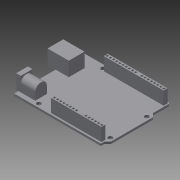
# Autodesk Inventor part: Arduino Uno
Saved by Autodesk Inventor 2015 (Build 190159000, 159)
## iProperties
Created: 2018-12-22
Part Number: Arduino Uno
Material: Типовые
Document SubType Name: Modeling
Designer: kostya
Density: 1 g/cm^3
Appearance: По умолчанию
Author: kostya
Autodesk Inventor part; units mm, degrees
ref_plane "YZ Plane" through (0, 0, 0) normal (1, 0, 0) x (0, 1, 0)
ref_plane "XZ Plane" through (0, 0, 0) normal (0, 1, 0) x (-1, 0, 0)
ref_plane "XY Plane" through (0, 0, 0) normal (0, 0, 1) x (1, 0, 0)
sketch "Эскиз1" plane through (0, 0, 0) normal (0, 0, 1) x (1, 0, 0)
  line L0 (-34.3, -26.6349) -> (31.8, -26.6349)
  line L1 (34.3, -21.3849) -> (34.3, 10.6851)
  line L2 (30.55, 26.6065) -> (-34.3, 26.6065)
  line L3 (-34.3, 26.6065) -> (-34.3, -26.6349)
  line L4 (-34.3, 26.6065) -> (-20.3, 26.6065) construction
  line L5 (-34.3, 26.6065) -> (16.5, 26.6065) construction
  line L6 (-34.3, 26.6065) -> (30.5, 26.6065) construction
  line L7 (34.3, 26.6065) -> (31.8, 26.6065) construction
  line L8 (-34.3, 26.6065) -> (-17, 26.6065) construction
  line L9 (-34.3, -26.6349) -> (-18.3, -26.6349) construction
  line L10 (-18.3, -26.6349) -> (-18.3, -25.4849) construction
  line L11 (-18.3, -25.4849) -> (-18.3, -22.2849) construction
  circle A0 centre (-18.3, -23.8849) radius 1.6
  line L12 (-17, 26.6065) -> (-17, 25.4565) construction
  line L13 (-17, 25.4565) -> (-17, 22.2565) construction
  circle A1 centre (-17, 23.8565) radius 1.6
  line L14 (34.3, -21.3849) -> (34.3, -19.1849) construction
  line L15 (34.3, -19.1849) -> (33.15, -19.1849) construction
  line L16 (33.15, -19.1849) -> (29.95, -19.1849) construction
  circle A2 centre (31.55, -19.1849) radius 1.6
  line L17 (31.55, -19.1849) -> (31.55, 8.7151) construction
  line L18 (31.55, 8.7151) -> (31.55, 10.3151) construction
  circle A3 centre (31.55, 8.7151) radius 1.6
  line L19 (-18.3, -23.8849) -> (34.3, -23.8849) construction
  line L20 (31.8, -23.8849) -> (34.3, -21.3849)
  line L21 (31.8, -23.8849) -> (34.3, -23.8849) construction
  line L22 (31.55, 10.3151) -> (31.55, 13.4351) construction
  line L23 (31.55, 13.4351) -> (34.3, 10.6851)
  line L24 (31.55, 13.4351) -> (35.4391, 13.4351) construction
  line L25 (31.55, 13.4351) -> (31.55, 25.6065)
  line L26 (31.8, -23.8849) -> (31.8, -26.6349)
  line L27 (31.55, 25.6065) -> (30.55, 26.6065)
  point P0 (0, 0)
  dimension "d0" = 68.6
  dimension "d7" = 17.3
  dimension "d8" = 16
  dimension "d9" = 1.15
  dimension "d10" = 3.2
  dimension "d11" = 1.15
  dimension "d12" = 3.2
  dimension "d13" = 4.7
  dimension "d14" = 1.15
  dimension "d15" = 3.2
  dimension "d18" = 27.9
  dimension "d19" = 1.6
  dimension "d20" = 45
  dimension "d21" = 3.12
  dimension "d22" = 45
  dimension "d25" = 53.2413
  constraints: 56 end point, 9 point on line, 6 horizontal, 4 vertical, 3 midpoint, 3 perpendicular, 3 vertical alignment, 2 parallel, 1 coincident, 1 equal length, 1 horizontal alignment, 8 other
  measures "d0" distance of L2.end L7.start
  measures "d7" distance of L2.end L8.end
  measures "d8" distance of L0.start L9.end
  measures "d9" distance of L9.end L10.end
  measures "d10" distance of L10.end L11.end
  measures "d11" distance of L8.end L12.end
  measures "d12" distance of L12.end L13.end
  measures "d13" distance of L19.end L14.end
  measures "d14" distance of L14.end L15.end
  measures "d15" distance of L15.end L16.end
  measures "d18" distance of L17.start L17.end
  measures "d19" distance of L17.end L18.end
  measures "d20" angle of L21 L20
  measures "d21" distance of L18.end L22.end
  measures "d22" angle of L23 L24
  measures "d25" distance of L7.end L0.end
extrude "Выдавливание1" add sketch "Эскиз1" along normal blind 1.6
sketch "Эскиз2" plane through (0, 0, 1.6) normal (0, 0, 1) x (1, 0, 0)
  circle A0 centre (31.55, 8.7151) radius 1.6 projected
  circle A1 centre (31.55, -19.1849) radius 1.6 projected
  circle A2 centre (-17, 23.8565) radius 1.6 projected
  circle A3 centre (-18.3, -23.8849) radius 1.6 projected
  line L0 (-34.3, -26.6349) -> (31.8, -26.6349) projected
  line L1 (31.8, -26.6349) -> (31.8, -23.8849) projected
  line L2 (31.8, -23.8849) -> (34.3, -21.3849) projected
  line L3 (34.3, -21.3849) -> (34.3, 10.6851) projected
  line L4 (34.3, 10.6851) -> (31.55, 13.4351) projected
  line L5 (31.55, 13.4351) -> (31.55, 25.6065) projected
  line L6 (31.55, 25.6065) -> (30.55, 26.6065) projected
  line L7 (30.55, 26.6065) -> (-34.3, 26.6065) projected
  line L8 (-34.3, 26.6065) -> (-34.3, -26.6349) projected
  line L9 (-34.3, 26.6065) -> (-34.3, 17.0065) construction
  line L10 (-34.3, 17.0065) -> (-40.5, 17.0065) construction
  line L11 (-40.5, 17.0065) -> (-40.5, 5.0065) construction
  line L12 (-40.5, 17.0065) -> (-24.3, 17.0065)
  line L13 (-24.3, 17.0065) -> (-24.3, 5.0065)
  line L14 (-24.3, 5.0065) -> (-40.5, 5.0065)
  line L15 (-40.5, 5.0065) -> (-40.5, 17.0065)
  line L16 (-34.3, -26.6349) -> (-34.3, -23.3349) construction
  line L17 (-34.3, 26.6065) -> (-34.3, -26.6349) construction
  line L18 (-34.3, -23.3349) -> (-36.1, -23.3349) construction
  line L19 (-36.1, -23.3349) -> (-36.1, -14.4349) construction
  line L20 (-36.1, -23.3349) -> (-21.6, -23.3349)
  line L21 (-21.6, -23.3349) -> (-21.6, -14.4349)
  line L22 (-21.6, -14.4349) -> (-36.1, -14.4349)
  line L23 (-36.1, -14.4349) -> (-36.1, -23.3349)
  point P0 (0, 0)
  dimension "d29" = 9.6
  dimension "d30" = 6.2
  dimension "d31" = 12
  dimension "d32" = 16.2
  dimension "d33" = 3.3
  dimension "d34" = 1.8
  dimension "d35" = 8.9
  dimension "d36" = 14.5
  constraints: 28 end point, 4 parallel, 4 perpendicular, 3 horizontal, 2 point on line, 1 vertical
  measures "d29" distance of L7.end L9.end
  measures "d30" distance of L9.end L10.end
  measures "d31" distance of L10.end L11.end
  measures "d32" distance of L13.end L14.end
  measures "d33" distance of L0.start L16.end
  measures "d34" distance of L16.end L18.end
  measures "d35" distance of L18.end L19.end
  measures "d36" distance of L22.end L21.end
extrude "Выдавливание2" add sketch "Эскиз2" along normal blind 10.9 contours L20 L23 L22 L8 | L8 L22 L21 L20 | L14 L15 L12 L8 | L8 L12 L13 L14
sketch "Эскиз3" plane through (-36.1, -23.3349, 1.6) normal (-1, 0, 0) x (0, 0, 1)
  line L0 (0, 8.9) -> (0, 0) projected
  line L1 (0, 0) -> (10.9, 0) projected
  line L2 (10.9, 8.9) -> (10.9, 0) projected
  line L3 (0, 8.9) -> (10.9, 8.9) projected
  line L4 (0, 8.9) -> (0, 0) projected
  line L5 (0, 4.45) -> (3.5, 4.45) construction
  line L6 (3.5, 4.45) -> (9.5, 4.45) construction
  circle A0 centre (6.5, 4.45) radius 3
  point P0 (-1.6, 23.3349)
  dimension "d39" = 3.5
  dimension "d40" = 6
  constraints: 4 end point, 2 horizontal, 2 midpoint, 1 horizontal alignment, 2 other
  measures "d39" distance of L5.start L5.end
  measures "d40" distance of L5.end L6.end
extrude "Выдавливание3" cut sketch "Эскиз3" against normal blind 9 contours A0
sketch "Эскиз4" plane through (-27.1, -18.8849, 8.1) normal (-1, 0, 0) x (0, 0, 1)
  circle A0 centre (0, 0) radius 0.5
  point P0 (-8.1, 18.8849)
  dimension "d43" = 1
  constraints: 1 centre point
  measures "d43" diameter of A0
extrude "Выдавливание4" add sketch "Эскиз4" along normal blind 9
fillet "Сопряжение1" radius 0.5 1 edges at (-36.1, -18.8849, 7.6)
sketch "Эскиз5" plane through (0, 0, 12.5) normal (0, 0, 1) x (1, 0, 0)
  line L0 (-36.1, -23.3349) -> (-21.6, -23.3349) projected
  line L1 (-21.6, -23.3349) -> (-21.6, -14.4349) projected
  line L2 (-21.6, -14.4349) -> (-36.1, -14.4349) projected
  line L3 (-36.1, -14.4349) -> (-36.1, -23.3349) projected
  line L4 (-36.1, -14.4349) -> (-32.6, -14.4349) construction
  line L5 (-21.6, -14.4349) -> (-36.1, -14.4349) construction
  line L6 (-32.6, -14.4349) -> (-32.6, -23.3349)
  line L7 (-36.1, -23.3349) -> (-21.6, -23.3349) projected
  line L8 (-36.1, -23.3349) -> (-32.6, -23.3349)
  line L9 (-36.1, -14.4349) -> (-36.1, -23.3349)
  line L10 (-36.1, -14.4349) -> (-32.6, -14.4349)
  point P0 (0, 0)
  dimension "d47" = 3.5
  constraints: 10 end point, 3 collinear, 2 point on line, 1 vertical
  measures "d47" distance of L2.end L4.end
extrude "Выдавливание5" cut sketch "Эскиз5" against normal blind 1 contours L6 L2 L1 L0
fillet "Сопряжение2" radius 4.25 2 edges at (-27.1, -23.3349, 11.5) (-27.1, -14.4349, 11.5)
sketch "Эскиз6" plane through (-40.5, 5.0065, 1.6) normal (-1, 0, 0) x (0, 0, 1)
  line L0 (0, 0) -> (0, 12) projected
  line L1 (0, 0) -> (10.9, 0) projected
  line L2 (10.9, 12) -> (10.9, 0) projected
  line L3 (0, 12) -> (10.9, 12) projected
  line L4 (10.9, 12) -> (10.9, 0) construction
  line L5 (10.9, 6) -> (0, 6) construction
  line L6 (0, 12) -> (0, 0) construction
  line L7 (0, 0) -> (10.9, 0) construction
  line L8 (5.45, 0) -> (5.45, 12) construction
  line L9 (3.85, 8.8) -> (7.05, 8.8)
  line L10 (7.05, 3.2) -> (3.85, 3.2)
  line L11 (3.85, 8.8) -> (7.05, 3.2) construction
  line L12 (7.05, 8.8) -> (3.85, 3.2) construction
  line L13 (0, 6) -> (1, 6) construction
  line L14 (1, 6) -> (1, 1.775)
  line L15 (1, 6) -> (1, 10.225)
  line L16 (1, 10.225) -> (6.9, 10.225)
  line L17 (8.9, 8.225) -> (8.9, 3.775)
  line L18 (6.9, 1.775) -> (1, 1.775)
  line L19 (7.8643, 10.225) -> (6.9, 10.225) construction
  line L20 (6.9, 10.225) -> (8.9, 8.225)
  line L21 (7.8643, 1.775) -> (6.9, 1.775) construction
  line L22 (6.9, 1.775) -> (8.9, 3.775)
  line L23 (6.9, 10.225) -> (6.9, 1.775) construction
  line L24 (8.9, 10.225) -> (6.9, 10.225) construction
  line L25 (7.05, 7.4) -> (5.45, 7.4) construction
  line L26 (7.05, 4.6) -> (5.45, 4.6) construction
  line L27 (7.05, 7.5) -> (6.9, 7.5) construction
  line L28 (7.05, 7.5) -> (6.9, 7.5)
  line L29 (6.9, 7.5) -> (6.9, 7.4)
  line L30 (6.9, 7.4) -> (6.9, 7.3)
  line L31 (6.9, 7.3) -> (7.05, 7.3)
  line L32 (6.9, 1.775) -> (6.9, 10.225) construction
  line L33 (7.05, 4.5) -> (6.9, 4.5) construction
  line L34 (7.05, 4.5) -> (6.9, 4.5)
  line L35 (6.9, 4.5) -> (6.9, 4.6)
  line L36 (6.9, 4.6) -> (6.9, 4.7)
  line L37 (6.9, 4.7) -> (7.05, 4.7)
  line L38 (4, 10.225) -> (4, 1.775) construction
  line L39 (3.85, 7.5) -> (4, 7.5) construction
  line L40 (3.85, 7.5) -> (4, 7.5)
  line L41 (4, 7.5) -> (4, 7.4)
  line L42 (4, 7.4) -> (4, 7.3)
  line L43 (4, 7.3) -> (3.85, 7.3)
  line L44 (4, 4.7) -> (3.85, 4.7)
  line L45 (4, 1.775) -> (4, 10.225) construction
  line L46 (4, 4.6) -> (4, 4.7)
  line L47 (4, 4.5) -> (4, 4.6)
  line L48 (3.85, 4.5) -> (4, 4.5) construction
  line L49 (3.85, 4.5) -> (4, 4.5)
  line L50 (7.05, 8.8) -> (7.05, 7.5)
  line L51 (7.05, 8.8) -> (7.05, 7.5) construction
  line L52 (7.05, 7.4) -> (7.05, 6) construction
  line L53 (7.05, 6) -> (7.05, 4.7) construction
  line L54 (7.05, 4.5) -> (7.05, 3.2) construction
  line L55 (7.05, 7.3) -> (7.05, 4.7)
  line L56 (7.05, 4.5) -> (7.05, 3.2)
  line L57 (3.85, 7.5) -> (3.85, 8.8)
  line L58 (3.85, 3.2) -> (3.85, 4.5)
  line L59 (3.85, 4.7) -> (3.85, 7.3)
  point P0 (-1.6, -5.0065)
  point P1 (5.45, 6)
  dimension "d51" = 3.2
  dimension "d52" = 5.6
  dimension "d53" = 1
  dimension "d54" = 4.225
  dimension "d55" = 4.225
  dimension "d56" = 7.9
  dimension "d58" = 45
  constraints: 106 end point, 21 symmetric about line, 19 point on line, 10 parallel, 10 perpendicular, 8 midpoint, 7 collinear, 4 vertical, 3 horizontal
  measures "d51" distance of L10.start L10.end
  measures "d52" distance of L9.end L10.start
  measures "d53" distance of L5.end L13.end
  measures "d54" distance of L13.end L14.end
  measures "d55" distance of L13.end L15.end
  measures "d56" distance of L15.end L24.start
  measures "d58" angle of L20 L19
extrude "Выдавливание6" cut sketch "Эскиз6" against normal blind 12 contours L15 L16 L20 L17 L22 L18 L14
sketch "Эскиз7" plane through (0, 0, 1.6) normal (0, 0, 1) x (1, 0, 0)
  line L0 (-24.3, 5.0065) -> (-34.3, 5.0065) projected
  line L1 (-34.3, 5.0065) -> (-34.3, -14.4349) projected
  line L2 (-34.3, -14.4349) -> (-21.6, -14.4349) projected
  line L3 (-21.6, -14.4349) -> (-21.6, -23.3349) projected
  line L4 (-21.6, -23.3349) -> (-34.3, -23.3349) projected
  line L5 (-34.3, -23.3349) -> (-34.3, -26.6349) projected
  line L6 (-34.3, -26.6349) -> (31.8, -26.6349) projected
  line L7 (31.8, -26.6349) -> (31.8, -23.8849) projected
  line L8 (31.8, -23.8849) -> (34.3, -21.3849) projected
  line L9 (34.3, -21.3849) -> (34.3, 10.6851) projected
  line L10 (34.3, 10.6851) -> (31.55, 13.4351) projected
  line L11 (31.55, 13.4351) -> (31.55, 25.6065) projected
  line L12 (31.55, 25.6065) -> (30.55, 26.6065) projected
  line L13 (30.55, 26.6065) -> (-34.3, 26.6065) projected
  line L14 (-34.3, 26.6065) -> (-34.3, 17.0065) projected
  line L15 (-34.3, 17.0065) -> (-24.3, 17.0065) projected
  line L16 (-24.3, 17.0065) -> (-24.3, 5.0065) projected
  circle A0 centre (31.55, 8.7151) radius 1.6 projected
  circle A1 centre (31.55, -19.1849) radius 1.6 projected
  circle A2 centre (-17, 23.8565) radius 1.6 projected
  circle A3 centre (-18.3, -23.8849) radius 1.6 projected
  line L17 (31.55, 13.4351) -> (31.55, 25.6065) construction
  circle A4 centre (-17, 23.8565) radius 1.6 construction
  line L18 (-15.4, 23.8565) -> (-14.9, 23.8565) construction
  line L19 (-14.9, 23.8565) -> (-14.9, 25.3565) construction
  line L20 (-14.9, 23.8565) -> (-14.9, 22.3565) construction
  line L21 (-14.9, 25.3565) -> (-12.5, 25.3565)
  line L22 (-12.5, 25.3565) -> (-12.5, 22.3565)
  line L23 (-12.5, 22.3565) -> (-14.9, 22.3565)
  line L24 (-14.9, 22.3565) -> (-14.9, 25.3565)
  line L25 (-14.4, 23.1565) -> (-13, 23.1565)
  line L26 (-13, 23.1565) -> (-13, 24.5565)
  line L27 (-13, 24.5565) -> (-14.4, 24.5565)
  line L28 (-14.4, 24.5565) -> (-14.4, 23.1565)
  line L29 (-14.4, 23.1565) -> (-13, 24.5565) construction
  line L30 (-13, 23.1565) -> (-14.4, 24.5565) construction
  point P0 (0, 0)
  point P1 (-13.7, 23.8565)
  dimension "d64" = 0.5
  dimension "d65" = 1.5
  dimension "d66" = 1.5
  dimension "d67" = 2.4
  dimension "d68" = 3
  dimension "d71" = 1.4
  dimension "d72" = 1.4
  constraints: 26 end point, 4 parallel, 2 horizontal, 2 midpoint, 2 perpendicular, 2 vertical, 1 horizontal alignment, 1 other
  measures "d64" distance of L18.start L18.end
  measures "d65" distance of L18.end L19.end
  measures "d66" distance of L18.end L20.end
  measures "d67" distance of L22.end L23.end
  measures "d68" distance of L21.end L22.end
  measures "d71" distance of L27.end L26.end
  measures "d72" distance of L26.end L25.end
extrude "Выдавливание7" add sketch "Эскиз7" along normal blind 10 contours L21 L22 L23 L24
pattern_linear "Прямоуг.массив1" count 19 spacing 2.4 along (1, 0, 0) of "Выдавливание7"
sketch "Эскиз8" plane through (0, 0, 1.6) normal (0, 0, 1) x (1, 0, 0)
  line L0 (9.6, 24.5565) -> (11, 24.5565)
  line L1 (11, 24.5565) -> (11, 23.1565)
  line L2 (11, 23.1565) -> (9.6, 23.1565)
  line L3 (9.6, 23.1565) -> (9.6, 24.5565)
  point P0 (0, 0)
  constraints: 8 end point, 2 parallel, 1 horizontal, 1 perpendicular
extrude "Выдавливание8" add sketch "Эскиз8" along normal blind 10
sketch "Эскиз9" plane through (0, 0, 1.6) normal (0, 0, 1) x (1, 0, 0)
  line L0 (30.7, 22.3565) -> (-14.9, 22.3565) projected
  line L1 (-14.9, 22.3565) -> (-14.9, 25.3565) projected
  line L2 (-14.9, 25.3565) -> (30.7, 25.3565) projected
  line L3 (30.7, 25.3565) -> (30.7, 22.3565) projected
  circle A0 centre (-18.3, -23.8849) radius 1.6 projected
  circle A1 centre (-17, 23.8565) radius 1.6 projected
  circle A2 centre (31.55, -19.1849) radius 1.6 projected
  circle A3 centre (31.55, 8.7151) radius 1.6 projected
  line L4 (-24.3, 5.0065) -> (-34.3, 5.0065) projected
  line L5 (-34.3, 5.0065) -> (-34.3, -14.4349) projected
  line L6 (-34.3, -14.4349) -> (-21.6, -14.4349) projected
  line L7 (-21.6, -14.4349) -> (-21.6, -23.3349) projected
  line L8 (-21.6, -23.3349) -> (-34.3, -23.3349) projected
  line L9 (-34.3, -23.3349) -> (-34.3, -26.6349) projected
  line L10 (-34.3, -26.6349) -> (31.8, -26.6349) projected
  line L11 (31.8, -26.6349) -> (31.8, -23.8849) projected
  line L12 (31.8, -23.8849) -> (34.3, -21.3849) projected
  line L13 (34.3, -21.3849) -> (34.3, 10.6851) projected
  line L14 (34.3, 10.6851) -> (31.55, 13.4351) projected
  line L15 (31.55, 13.4351) -> (31.55, 25.6065) projected
  line L16 (31.55, 25.6065) -> (30.55, 26.6065) projected
  line L17 (30.55, 26.6065) -> (-34.3, 26.6065) projected
  line L18 (-34.3, 26.6065) -> (-34.3, 17.0065) projected
  line L19 (-34.3, 17.0065) -> (-24.3, 17.0065) projected
  line L20 (-24.3, 17.0065) -> (-24.3, 5.0065) projected
  line L21 (31.8, -26.6349) -> (30.95, -26.6349) construction
  line L22 (-34.3, -26.6349) -> (31.8, -26.6349) construction
  line L23 (30.95, -26.6349) -> (30.95, -25.3849) construction
  line L24 (-14.9, 25.3565) -> (-14.9, 22.3565) projected
  line L25 (30.7, 25.3565) -> (-14.9, 25.3565) projected
  line L26 (-12, 23.1565) -> (-12, 24.5565) projected
  line L27 (-12, 24.5565) -> (-10.6, 24.5565) projected
  line L28 (-10.6, 24.5565) -> (-10.6, 23.1565) projected
  line L29 (-10.6, 23.1565) -> (-12, 23.1565) projected
  line L30 (-9.6, 23.1565) -> (-9.6, 24.5565) projected
  line L31 (-9.6, 24.5565) -> (-8.2, 24.5565) projected
  line L32 (-8.2, 24.5565) -> (-8.2, 23.1565) projected
  line L33 (-8.2, 23.1565) -> (-9.6, 23.1565) projected
  line L34 (-7.2, 23.1565) -> (-7.2, 24.5565) projected
  line L35 (-7.2, 24.5565) -> (-5.8, 24.5565) projected
  line L36 (-5.8, 24.5565) -> (-5.8, 23.1565) projected
  line L37 (-5.8, 23.1565) -> (-7.2, 23.1565) projected
  line L38 (-4.8, 23.1565) -> (-4.8, 24.5565) projected
  line L39 (-4.8, 24.5565) -> (-3.4, 24.5565) projected
  line L40 (-3.4, 24.5565) -> (-3.4, 23.1565) projected
  line L41 (-3.4, 23.1565) -> (-4.8, 23.1565) projected
  line L42 (-2.4, 23.1565) -> (-2.4, 24.5565) projected
  line L43 (-2.4, 24.5565) -> (-1, 24.5565) projected
  line L44 (-1, 24.5565) -> (-1, 23.1565) projected
  line L45 (-1, 23.1565) -> (-2.4, 23.1565) projected
  line L46 (0, 23.1565) -> (0, 24.5565) projected
  line L47 (0, 24.5565) -> (1.4, 24.5565) projected
  line L48 (1.4, 24.5565) -> (1.4, 23.1565) projected
  line L49 (1.4, 23.1565) -> (0, 23.1565) projected
  line L50 (2.4, 23.1565) -> (2.4, 24.5565) projected
  line L51 (2.4, 24.5565) -> (3.8, 24.5565) projected
  line L52 (3.8, 24.5565) -> (3.8, 23.1565) projected
  line L53 (3.8, 23.1565) -> (2.4, 23.1565) projected
  line L54 (4.8, 23.1565) -> (4.8, 24.5565) projected
  line L55 (4.8, 24.5565) -> (6.2, 24.5565) projected
  line L56 (6.2, 24.5565) -> (6.2, 23.1565) projected
  line L57 (6.2, 23.1565) -> (4.8, 23.1565) projected
  line L58 (7.2, 23.1565) -> (7.2, 24.5565) projected
  line L59 (7.2, 24.5565) -> (8.6, 24.5565) projected
  line L60 (8.6, 24.5565) -> (8.6, 23.1565) projected
  line L61 (8.6, 23.1565) -> (7.2, 23.1565) projected
  line L62 (12, 23.1565) -> (12, 24.5565) projected
  line L63 (12, 24.5565) -> (13.4, 24.5565) projected
  line L64 (13.4, 24.5565) -> (13.4, 23.1565) projected
  line L65 (13.4, 23.1565) -> (12, 23.1565) projected
  line L66 (14.4, 23.1565) -> (14.4, 24.5565) projected
  line L67 (14.4, 24.5565) -> (15.8, 24.5565) projected
  line L68 (15.8, 24.5565) -> (15.8, 23.1565) projected
  line L69 (15.8, 23.1565) -> (14.4, 23.1565) projected
  line L70 (16.8, 23.1565) -> (16.8, 24.5565) projected
  line L71 (16.8, 24.5565) -> (18.2, 24.5565) projected
  line L72 (18.2, 24.5565) -> (18.2, 23.1565) projected
  line L73 (18.2, 23.1565) -> (16.8, 23.1565) projected
  line L74 (19.2, 23.1565) -> (19.2, 24.5565) projected
  line L75 (19.2, 24.5565) -> (20.6, 24.5565) projected
  line L76 (20.6, 24.5565) -> (20.6, 23.1565) projected
  line L77 (20.6, 23.1565) -> (19.2, 23.1565) projected
  line L78 (21.6, 23.1565) -> (21.6, 24.5565) projected
  line L79 (21.6, 24.5565) -> (23, 24.5565) projected
  line L80 (23, 24.5565) -> (23, 23.1565) projected
  line L81 (23, 23.1565) -> (21.6, 23.1565) projected
  line L82 (24, 23.1565) -> (24, 24.5565) projected
  line L83 (24, 24.5565) -> (25.4, 24.5565) projected
  line L84 (25.4, 24.5565) -> (25.4, 23.1565) projected
  line L85 (25.4, 23.1565) -> (24, 23.1565) projected
  line L86 (26.4, 23.1565) -> (26.4, 24.5565) projected
  line L87 (26.4, 24.5565) -> (27.8, 24.5565) projected
  line L88 (27.8, 24.5565) -> (27.8, 23.1565) projected
  line L89 (27.8, 23.1565) -> (26.4, 23.1565) projected
  line L90 (28.8, 23.1565) -> (28.8, 24.5565) projected
  line L91 (28.8, 24.5565) -> (30.2, 24.5565) projected
  line L92 (30.2, 24.5565) -> (30.2, 23.1565) projected
  line L93 (30.2, 23.1565) -> (28.8, 23.1565) projected
  line L94 (-14.4, 23.1565) -> (-14.4, 24.5565) projected
  line L95 (-14.4, 24.5565) -> (-13, 24.5565) projected
  line L96 (-13, 24.5565) -> (-13, 23.1565) projected
  line L97 (-13, 23.1565) -> (-14.4, 23.1565) projected
  line L98 (30.7, 25.3565) -> (-14.9, 25.3565) projected
  line L99 (-14.9, 25.3565) -> (-14.9, 22.3565) projected
  line L100 (-14.9, 22.3565) -> (30.7, 22.3565) projected
  line L101 (30.7, 22.3565) -> (30.7, 25.3565) projected
  line L102 (30.95, -25.3849) -> (28.55, -25.3849)
  line L103 (28.55, -25.3849) -> (28.55, -22.3849)
  line L104 (28.55, -22.3849) -> (30.95, -22.3849)
  line L105 (30.95, -22.3849) -> (30.95, -25.3849)
  line L106 (29.05, -24.5849) -> (30.45, -24.5849)
  line L107 (30.45, -24.5849) -> (30.45, -23.1849)
  line L108 (30.45, -23.1849) -> (29.05, -23.1849)
  line L109 (29.05, -23.1849) -> (29.05, -24.5849)
  line L110 (29.05, -24.5849) -> (30.45, -23.1849) construction
  line L111 (30.45, -24.5849) -> (29.05, -23.1849) construction
  point P0 (0, 0)
  point P1 (29.75, -23.8849)
  dimension "d80" = 0.85
  dimension "d81" = 1.25
  dimension "d82" = 2.4
  dimension "d83" = 3
  dimension "d84" = 1.4
  dimension "d85" = 1.4
  constraints: 24 end point, 4 parallel, 2 horizontal, 2 midpoint, 2 perpendicular, 1 point on line, 1 vertical
  measures "d80" distance of L10.end L21.end
  measures "d81" distance of L21.end L23.end
  measures "d82" distance of L103.end L104.end
  measures "d83" distance of L102.end L103.end
  measures "d84" distance of L108.end L107.end
  measures "d85" distance of L107.end L106.end
extrude "Выдавливание9" add sketch "Эскиз9" along normal blind 10 contours L102 L103 L104 L105
pattern_linear "Прямоуг.массив2" count 16 spacing 2.4 along (-1, 0, 0) of "Выдавливание9"
sketch "Эскиз10" plane through (0, 0, 1.6) normal (0, 0, 1) x (1, 0, 0)
  line L0 (26.65, -24.5849) -> (26.65, -23.1849) projected
  line L1 (26.65, -23.1849) -> (28.05, -23.1849) projected
  line L2 (28.05, -23.1849) -> (28.05, -24.5849) projected
  line L3 (28.05, -24.5849) -> (26.65, -24.5849) projected
  line L4 (24.25, -24.5849) -> (24.25, -23.1849) projected
  line L5 (24.25, -23.1849) -> (25.65, -23.1849) projected
  line L6 (25.65, -23.1849) -> (25.65, -24.5849) projected
  line L7 (25.65, -24.5849) -> (24.25, -24.5849) projected
  line L8 (21.85, -24.5849) -> (21.85, -23.1849) projected
  line L9 (21.85, -23.1849) -> (23.25, -23.1849) projected
  line L10 (23.25, -23.1849) -> (23.25, -24.5849) projected
  line L11 (23.25, -24.5849) -> (21.85, -24.5849) projected
  line L12 (19.45, -24.5849) -> (19.45, -23.1849) projected
  line L13 (19.45, -23.1849) -> (20.85, -23.1849) projected
  line L14 (20.85, -23.1849) -> (20.85, -24.5849) projected
  line L15 (20.85, -24.5849) -> (19.45, -24.5849) projected
  line L16 (17.05, -24.5849) -> (17.05, -23.1849) projected
  line L17 (17.05, -23.1849) -> (18.45, -23.1849) projected
  line L18 (18.45, -23.1849) -> (18.45, -24.5849) projected
  line L19 (18.45, -24.5849) -> (17.05, -24.5849) projected
  line L20 (14.65, -24.5849) -> (14.65, -23.1849) projected
  line L21 (14.65, -23.1849) -> (16.05, -23.1849) projected
  line L22 (16.05, -23.1849) -> (16.05, -24.5849) projected
  line L23 (16.05, -24.5849) -> (14.65, -24.5849) projected
  line L24 (12.25, -24.5849) -> (12.25, -23.1849) projected
  line L25 (12.25, -23.1849) -> (13.65, -23.1849) projected
  line L26 (13.65, -23.1849) -> (13.65, -24.5849) projected
  line L27 (13.65, -24.5849) -> (12.25, -24.5849) projected
  line L28 (9.85, -24.5849) -> (9.85, -23.1849) projected
  line L29 (9.85, -23.1849) -> (11.25, -23.1849) projected
  line L30 (11.25, -23.1849) -> (11.25, -24.5849) projected
  line L31 (11.25, -24.5849) -> (9.85, -24.5849) projected
  line L32 (7.45, -24.5849) -> (7.45, -23.1849) projected
  line L33 (7.45, -23.1849) -> (8.85, -23.1849) projected
  line L34 (8.85, -23.1849) -> (8.85, -24.5849) projected
  line L35 (8.85, -24.5849) -> (7.45, -24.5849) projected
  line L36 (5.05, -24.5849) -> (5.05, -23.1849) projected
  line L37 (5.05, -23.1849) -> (6.45, -23.1849) projected
  line L38 (6.45, -23.1849) -> (6.45, -24.5849) projected
  line L39 (6.45, -24.5849) -> (5.05, -24.5849) projected
  line L40 (2.65, -24.5849) -> (2.65, -23.1849) projected
  line L41 (2.65, -23.1849) -> (4.05, -23.1849) projected
  line L42 (4.05, -23.1849) -> (4.05, -24.5849) projected
  line L43 (4.05, -24.5849) -> (2.65, -24.5849) projected
  line L44 (0.25, -24.5849) -> (0.25, -23.1849) projected
  line L45 (0.25, -23.1849) -> (1.65, -23.1849) projected
  line L46 (1.65, -23.1849) -> (1.65, -24.5849) projected
  line L47 (1.65, -24.5849) -> (0.25, -24.5849) projected
  line L48 (-2.15, -24.5849) -> (-2.15, -23.1849) projected
  line L49 (-2.15, -23.1849) -> (-0.75, -23.1849) projected
  line L50 (-0.75, -23.1849) -> (-0.75, -24.5849) projected
  line L51 (-0.75, -24.5849) -> (-2.15, -24.5849) projected
  line L52 (-4.55, -24.5849) -> (-4.55, -23.1849) projected
  line L53 (-4.55, -23.1849) -> (-3.15, -23.1849) projected
  line L54 (-3.15, -23.1849) -> (-3.15, -24.5849) projected
  line L55 (-3.15, -24.5849) -> (-4.55, -24.5849) projected
  line L56 (-6.95, -24.5849) -> (-6.95, -23.1849) projected
  line L57 (-6.95, -23.1849) -> (-5.55, -23.1849) projected
  line L58 (-5.55, -23.1849) -> (-5.55, -24.5849) projected
  line L59 (-5.55, -24.5849) -> (-6.95, -24.5849) projected
  line L60 (29.05, -24.5849) -> (29.05, -23.1849) projected
  line L61 (29.05, -23.1849) -> (30.45, -23.1849) projected
  line L62 (30.45, -23.1849) -> (30.45, -24.5849) projected
  line L63 (30.45, -24.5849) -> (29.05, -24.5849) projected
  line L64 (-7.45, -25.3849) -> (30.95, -25.3849) projected
  line L65 (30.95, -25.3849) -> (30.95, -22.3849) projected
  line L66 (30.95, -22.3849) -> (-7.45, -22.3849) projected
  line L67 (-7.45, -22.3849) -> (-7.45, -25.3849) projected
  line L68 (16.05, -24.5849) -> (14.65, -24.5849)
  line L69 (14.65, -24.5849) -> (14.65, -23.1849)
  line L70 (14.65, -23.1849) -> (16.05, -23.1849)
  line L71 (16.05, -23.1849) -> (16.05, -24.5849)
  line L72 (16.05, -24.5849) -> (14.65, -23.1849) construction
  line L73 (14.65, -24.5849) -> (16.05, -23.1849) construction
  line L74 (13.65, -24.5849) -> (12.25, -24.5849)
  line L75 (12.25, -24.5849) -> (12.25, -23.1849)
  line L76 (12.25, -23.1849) -> (13.65, -23.1849)
  line L77 (13.65, -23.1849) -> (13.65, -24.5849)
  line L78 (13.65, -24.5849) -> (12.25, -23.1849) construction
  line L79 (12.25, -24.5849) -> (13.65, -23.1849) construction
  point P0 (0, 0)
  point P1 (15.35, -23.8849)
  point P2 (12.95, -23.8849)
  constraints: 24 end point, 4 midpoint, 4 parallel, 2 horizontal, 2 perpendicular
extrude "Выдавливание10" add sketch "Эскиз10" along normal blind 10 contours L20 L21 L22 L23 | L24 L25 L26 L27
